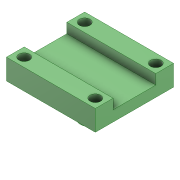
# Autodesk Inventor part: 지름 모터 커버
Saved by Autodesk Inventor 2020 (Build 240168000, 168)
## iProperties
Created: 2020-05-07
Part Number: 지름 모터 커버
Material: 일반
Document SubType Name: Modeling
Designer: sbahn
Density: 1 g/cm^3
Appearance: 매끄러움 - 짙은 산림 녹색
Author: sbahn
## iProperties of the stored document _3D 인쇄.ipt
Created: 2020-06-04
Part Number: _3D 인쇄
Material: 일반
Document SubType Name: Modeling
Designer: Miji
Density: 1 g/cm^3
Appearance: 기본값
Author: Miji
Autodesk Inventor part; units mm, degrees
ref_plane "YZ Plane" through (0, 0, 0) normal (1, 0, 0) x (0, 1, 0)
ref_plane "XZ Plane" through (0, 0, 0) normal (0, 1, 0) x (-1, 0, 0)
ref_plane "XY Plane" through (0, 0, 0) normal (0, 0, 1) x (1, 0, 0)
sketch "스케치1" plane through (0, 0, 0) normal (0, 1, 0) x (-1, 0, 0)
  line L0 (0, 0) -> (25, 0)
  line L1 (25, 0) -> (25, -22)
  line L2 (25, -22) -> (0, -22)
  line L3 (0, -22) -> (0, 0)
  dimension "d0" = 25
  dimension "d1" = 22
  constraints: 8 end point, 2 parallel, 1 horizontal, 1 perpendicular
  measures "d0" distance of L1.end L2.end
  measures "d1" distance of L0.end L1.end
extrude "돌출1" add sketch "스케치1" along normal blind 3
sketch "스케치2" plane through (0, 3, 0) normal (0, 1, 0) x (1, 0, 0)
  line L0 (0, 0) -> (0, 22) projected
  line L1 (0, 22) -> (-25, 22) projected
  line L2 (-25, 22) -> (-25, 0) projected
  line L3 (-25, 0) -> (0, 0) projected
  line L4 (-25, 0) -> (0, 0)
  line L5 (0, 0) -> (0, 5)
  line L6 (0, 5) -> (-25, 5)
  line L7 (-25, 5) -> (-25, 0)
  line L8 (-25, 22) -> (0, 22)
  line L9 (0, 22) -> (0, 17)
  line L10 (0, 17) -> (-25, 17)
  line L11 (-25, 17) -> (-25, 22)
  dimension "d4" = 5
  dimension "d5" = 5
  constraints: 16 end point, 4 parallel, 2 horizontal, 2 perpendicular, 2 point on line
  measures "d4" distance between parallel lines of L1 L10
  measures "d5" distance between parallel lines of L3 L6
extrude "돌출2" add sketch "스케치2" along normal blind 2.8 contours L3 L2 L6 L0 | L10 L2 L1 L0
sketch "스케치3" plane through (0, 0, 0) normal (0, -1, 0) x (1, 0, 0)
  line L0 (0, 0) -> (0, -22) projected
  line L1 (-25, 0) -> (0, 0) projected
  line L2 (-25, -22) -> (-25, 0) projected
  line L3 (0, -22) -> (-25, -22) projected
  line L4 (-22.5, -19.5) -> (-22.5, -2.5)
  line L5 (-22.5, -2.5) -> (-2.5, -2.5)
  line L6 (-2.5, -2.5) -> (-2.5, -19.5)
  line L7 (-2.5, -19.5) -> (-22.5, -19.5)
  dimension "d8" = 2.5
  constraints: 8 end point, 4 coincident, 3 other
  measures "d8" distance between parallel lines of L3 L7
hole "구멍1" at (-2.5, 0, -19.5) at (-2.5, 0, -2.5) at (-22.5, 0, -2.5) at (-22.5, 0, -19.5) direction (0, 1, 0) diameter 3 depth 8 tip angle 118 countersink diameter 4.5 countersink angle 90
sketch "스케치4" plane through (0, 0, 0) normal (0, -1, 0) x (1, 0, 0)
  circle A0 centre (-22.5, -2.5) radius 2.25 projected
  circle A1 centre (-2.5, -19.5) radius 2.25 projected
  circle A2 centre (-2.5, -2.5) radius 2.25 projected
  circle A3 centre (-22.5, -19.5) radius 2.25 projected
  line L0 (-25, 0) -> (0, 0) projected
  line L1 (-25, -22) -> (-25, 0) projected
  line L2 (0, -22) -> (-25, -22) projected
  line L3 (0, 0) -> (0, -22) projected
  circle A4 centre (-12.72, -11) radius 2.5
  dimension "d16" = 5
  dimension "d20" = 12.72
  constraints: 1 centre point
  measures "d16" diameter of A4
  measures "d20" distance from line of L3 A4.centre
extrude "돌출3" add sketch "스케치4" along normal blind 8.7 contours A4
sketch "스케치5" plane through (-12.72, -8.7, -11) normal (0, -1, 0) x (1, 0, 0)
  circle A0 centre (0, 0) radius 2.5 projected
  circle A1 centre (0, 0) radius 1.25
  point P0 (12.72, 11)
  dimension "d19" = 2.5
  constraints: 1 centre point, 1 coincident
  measures "d19" diameter of A1
extrude "돌출4" cut sketch "스케치5" against normal blind 7.05 contours A1
fillet "모깎기1" radius 2 1 edges at (-15.22, 0, -11)
